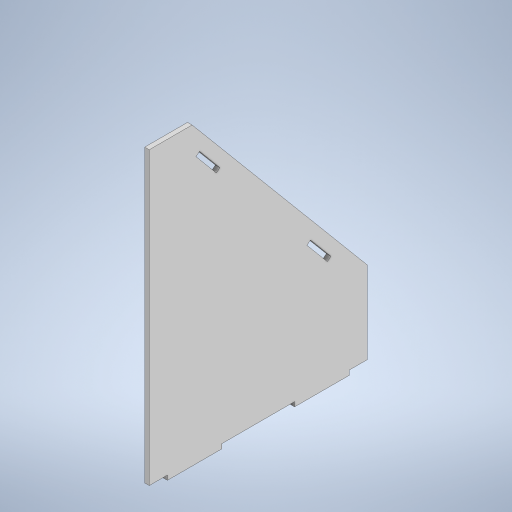
# Autodesk Inventor part: C4Side
Saved by Autodesk Inventor 2024 (Build 280153000, 153)
## iProperties
Created: 2023-11-07
Part Number: C4Side
Material: Generic
Document SubType Name: Modeling
Designer: flynf
Density: 1 g/cm^3
Appearance: Default
Author: flynf
Autodesk Inventor part; units mm, degrees
ref_plane "YZ Plane" through (0, 0, 0) normal (1, 0, 0) x (0, 1, 0)
ref_plane "XZ Plane" through (0, 0, 0) normal (0, 1, 0) x (-1, 0, 0)
ref_plane "XY Plane" through (0, 0, 0) normal (0, 0, 1) x (1, 0, 0)
sketch "Sketch2" plane through (0, 0, 0) normal (1, 0, 0) x (0, 1, 0)
  line L0 (0, 0) -> (0, -12.7)
  line L1 (0, -12.7) -> (-3.175, -12.7)
  line L2 (-3.175, -12.7) -> (-3.175, -50.8)
  line L3 (-3.175, -50.8) -> (0, -50.8)
  line L4 (0, -50.8) -> (0, -101.6)
  line L5 (0, -101.6) -> (-3.175, -101.6)
  line L6 (-3.175, -101.6) -> (-3.175, -139.7)
  line L7 (-3.175, -139.7) -> (0, -139.7)
  line L8 (0, -139.7) -> (0, -152.4)
  line L9 (0, 0) -> (203.2, 0)
  line L10 (203.2, -29.949) -> (57.2685, -152.4)
  line L11 (203.2, -29.949) -> (203.2, 0)
  line L12 (0, -152.4) -> (57.2685, -152.4)
  dimension "d18" = 12.7
  dimension "d19" = 3.175
  dimension "d20" = 38.1
  dimension "d21" = 3.175
  dimension "d22" = 50.8
  dimension "d23" = 3.175
  dimension "d24" = 38.1
  dimension "d25" = 3.175
  dimension "d26" = 12.7
  dimension "d27" = 203.2
  dimension "d28" = 190.5
  dimension "d29" = 90
  dimension "d30" = -130
  dimension "d31" = 0
  constraints: 26 end point, 5 perpendicular, 2 horizontal, 2 point on line, 1 vertical
  measures "d18" distance of L0.start L0.end
  measures "d19" distance of L0.end L1.end
  measures "d20" distance of L1.end L2.end
  measures "d21" distance of L2.end L3.end
  measures "d22" distance of L3.end L4.end
  measures "d23" distance of L4.end L5.end
  measures "d24" distance of L5.end L6.end
  measures "d25" distance of L6.end L7.end
  measures "d26" distance of L7.end L8.end
  measures "d27" distance of L0.start L9.end
  measures "d28" distance of L10.start L10.end
  measures "d29" angle of L9 L11
  measures "d30" angle of L11 L10
  measures "d31" vertical distance of L8.end L10.end
extrude "Extrusion2" add sketch "Sketch2" along normal blind 3.175
sketch "Sketch3" plane through (3.175, 0, 0) normal (1, 0, 0) x (0, 0, -1)
  line L0 (152.4, 57.2685) -> (29.949, 203.2) projected
  line L1 (152.4, 57.2685) -> (137.8069, 45.0234)
  line L2 (137.8069, 45.0234) -> (15.3558, 190.9549)
  line L3 (15.3558, 190.9549) -> (29.949, 203.2)
  line L4 (146.3195, 52.1664) -> (23.8685, 198.0979)
  line L5 (143.8873, 50.1256) -> (21.4363, 196.057)
  line L6 (32.661, 182.68) -> (35.0932, 184.7208)
  line L7 (46.9469, 165.6546) -> (49.3791, 167.6955)
  line L8 (110.2133, 90.2567) -> (112.6455, 92.2976)
  line L9 (124.4992, 73.2314) -> (126.9314, 75.2722)
  point P0 (0, 0)
  dimension "d34" = 19.05
  dimension "d35" = 3.175
  dimension "d36" = 7.9375
  dimension "d37" = 17.4625
  dimension "d38" = 22.225
  dimension "d39" = 98.425
  dimension "d40" = 22.225
  constraints: 18 end point, 12 point on line, 9 perpendicular
  measures "d34" distance between parallel lines of L0 L2
  measures "d35" distance between parallel lines of L4 L5
  measures "d36" distance between parallel lines of L0 L4
  measures "d37" distance between parallel lines of L3 L6
  measures "d38" distance between parallel lines of L6 L7
  measures "d39" distance between parallel lines of L7 L8
  measures "d40" distance between parallel lines of L8 L9
extrude "Extrusion3" cut sketch "Sketch3" against normal blind 3.175 contours L9 L5 L8 L4 | L4 L7 L5 L6
body "Solid2"
